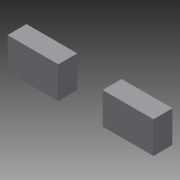
# Autodesk Inventor part: BumperFront
Saved by Autodesk Inventor 2013 (Build 170138000, 138)
## iProperties
Created: 2014-01-09
Part Number: BumperFront
Material: Generic
Document SubType Name: Modeling
Designer: 215152
Density: 1 g/cm^3
Author: 215152
Autodesk Inventor part; units mm, degrees
ref_plane "YZ Plane" through (0, 0, 0) normal (1, 0, 0) x (0, 1, 0)
ref_plane "XZ Plane" through (0, 0, 0) normal (0, 1, 0) x (-1, 0, 0)
ref_plane "XY Plane" through (0, 0, 0) normal (0, 0, 1) x (1, 0, 0)
sketch "Sketch1" plane through (0, 0, 0) normal (0, 0, 1) x (1, 0, 0)
  line L0 (0, 0) -> (-92.075, 0)
  line L1 (-92.075, 0) -> (-92.075, -101.6)
  line L2 (-92.075, -101.6) -> (-92.075, 25.4)
  line L3 (-92.075, 25.4) -> (492.125, 25.4)
  line L4 (492.125, 25.4) -> (492.125, -101.6)
  line L5 (492.125, -101.6) -> (-92.075, -101.6)
  dimension "d0" = 92.075
  dimension "d1" = 101.6
  dimension "d2" = 127
  dimension "d3" = 584.2
  dimension "d4" = 127
  constraints: 12 end point, 2 perpendicular, 1 collinear, 1 horizontal, 1 parallel
  measures "d0" distance of L0.start L0.end
  measures "d1" distance of L0.end L1.end
  measures "d2" distance of L1.end L2.end
  measures "d3" distance of L2.end L3.end
  measures "d4" distance of L3.end L4.end
extrude "Extrusion1" add sketch "Sketch1" along normal blind 76.2
sketch "Sketch2" plane through (-92.075, -101.6, 0) normal (0, -1, 0) x (1, 0, 0)
  line L0 (584.2, 0) -> (0, 0) projected
  line L1 (584.2, 0) -> (584.2, 76.2) projected
  line L2 (0, 76.2) -> (584.2, 76.2) projected
  line L3 (0, 0) -> (0, 76.2) projected
  line L4 (0, 76.2) -> (203.2, 76.2)
  line L5 (203.2, 76.2) -> (203.2, 0)
  line L6 (203.2, 0) -> (0, 0)
  line L7 (0, 0) -> (0, 76.2)
  line L8 (584.2, 0) -> (381, 0)
  line L9 (381, 0) -> (381, 76.2)
  line L10 (381, 76.2) -> (584.2, 76.2)
  line L11 (584.2, 76.2) -> (584.2, 0)
  point P0 (92.075, 0)
  dimension "d7" = 203.2
  dimension "d8" = 203.2
  dimension "d9" = 76.2
  constraints: 16 end point, 4 parallel, 2 horizontal, 2 perpendicular, 1 point on line
  measures "d7" distance of L5.end L6.end
  measures "d8" distance of L9.end L10.end
  measures "d9" distance of L8.end L9.end
extrude "Extrusion2" cut sketch "Sketch2" against normal blind 127 contours L0 L5 L2 L9
body "Solid1"
